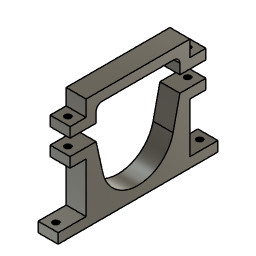
CuadroMediana (Autodesk Fusion 360 design; units mm, degrees)
Autodesk Fusion 360 part; units mm, degrees
sketch "Boceto1" plane through (0, 0, 0) normal (1, 0, 0) x (0, 1, 0)
  line L0 (-17.9997, 45.5) -> (18.0008, 45.5)
  line L1 (21.0003, 42.5) -> (21.0003, 37.5)
  line L2 (21.0003, 37.5) -> (-20.9997, 37.5)
  line L3 (-20.9997, 37.5) -> (-20.9997, 42.5)
  line L4 (-25.9997, 50.5) -> (26.0003, 50.5)
  line L5 (26.0003, 50.5) -> (26.0003, 42.5)
  line L6 (24, 37.5) -> (-27.0128, 37.5)
  line L7 (-25.9997, 42.5) -> (-25.9997, 50.5)
  line L8 (24, 37.5) -> (34.0003, 37.5)
  line L9 (34.0003, 37.5) -> (34.0003, 42.5)
  line L10 (34.0003, 42.5) -> (26.0003, 42.5)
  line L11 (-27.0128, 37.5) -> (-33.9997, 37.5)
  line L12 (-33.9997, 37.5) -> (-33.9997, 42.5)
  line L13 (-33.9997, 42.5) -> (-25.9997, 42.5)
  line L14 (-72.816, 37.5) -> (66.1059, 37.5)
  line L15 (21.0003, 37.5) -> (17.5697, 22.0889)
  line L16 (-20.9997, 37.5) -> (-17.5704, 22.09)
  arc A0 (-17.5704, 22.09) -> (17.5697, 22.0889) centre (-0.0002, 26) ccw
  line L17 (-33.9997, 37.5) -> (-23.996, 37.5)
  line L18 (-25.9997, 32.5) -> (-33.9997, 32.5)
  line L19 (-33.9997, 32.5) -> (-33.9997, 37.5)
  line L20 (24, 37.5) -> (34.0003, 37.5)
  line L21 (34.0003, 37.5) -> (34.0003, 32.5)
  line L22 (34.0003, 32.5) -> (26.0003, 32.5)
  line L23 (-25.9997, 32.5) -> (-25.9997, 7.5)
  line L24 (-25.9997, 7.5) -> (-40, 7.5)
  line L25 (-40, 7.5) -> (-40, 2.5)
  line L26 (-40, 2.5) -> (40.0003, 2.5)
  line L27 (40.0003, 2.5) -> (40.0003, 7.5)
  line L28 (40.0003, 7.5) -> (26.0003, 7.5)
  line L29 (26.0003, 7.5) -> (26.0003, 32.5)
  line L30 (-0.0002, 36.8459) -> (-0.0002, 16.8459)
  arc A1 (-17.9997, 45.5) -> (-20.9997, 42.5) centre (-17.9997, 42.5) ccw
  arc A2 (21.0003, 42.5) -> (17.9998, 45.5) centre (18.0003, 42.5) ccw
  dimension "d3" = 52
  dimension "d6" = 5
  dimension "d8" = 5
  dimension "d13" = 18
  dimension "d16" = 5
  dimension "d18" = 5
  dimension "d19" = 14
  dimension "d20" = 5
  dimension "d23" = 25
  dimension "d25" = 90
  dimension "d26" = 5
  dimension "d27" = 11.5
  dimension "d31" = 3
  dimension "d32" = 3
  dimension "d51" = 42
  dimension "d52" = 5
  dimension "d53" = 8
  dimension "d54" = 8
  dimension "d55" = 52
  dimension "d56" = 8
  dimension "d57" = 13
  dimension "d58" = 8
  dimension "d59" = 14.0003
  dimension "d60" = 8
  constraint horizontal L0
  constraint vertical L1
  constraint horizontal L2
  constraint vertical L3
  constraint horizontal L4
  constraint vertical L5
  constraint horizontal L6
  constraint vertical L7
  constraint horizontal L8
  constraint vertical L9
  constraint horizontal L10
  constraint horizontal L11
  constraint vertical L12
  constraint horizontal L13
  constraint perpendicular L12 L14
  constraint tangent L15 A0
  constraint tangent L16 A0
  constraint horizontal L17
  constraint horizontal L18
  constraint vertical L19
  constraint horizontal L20
  constraint vertical L21
  constraint horizontal L22
  constraint perpendicular L18 L23
  constraint perpendicular L23 L24
  constraint perpendicular L18 L25
  constraint perpendicular L25 L26
  constraint perpendicular L26 L27
  constraint perpendicular L22 L29
  constraint perpendicular L14 L30
  constraint coincident A0.centre L30
  constraint coincident L2.end L14
  constraint coincident L14 L17.end
  constraint tangent L3 A1
  constraint tangent L0 A1
  constraint coincident L0.start A1
  constraint coincident L0 A1.start
  constraint coincident L0.end A2
  constraint tangent L1 A2
  constraint coincident L0 A2.end
  measures "d3" distance of L4.start L4.end
  measures "d6" distance of L8.end L9.end
  measures "d8" distance of L11.end L12.end
  measures "d13" radius of A0
  measures "d16" distance of L11.end L18.end
  measures "d18" distance of L8.end L21.end
  measures "d19" distance of L27.end L28.end
  measures "d20" distance of L26.end L27.end
  measures "d23" distance of L22.end L28.end
  measures "d25" angle of L28 L29
  measures "d26" distance of L24.end L25.end
  measures "d27" distance of L14 A0.centre
  measures "d31" radius of A1
  measures "d32" radius of A2
  measures "d51" distance of L1 L3
  measures "d52" distance of L1 L5
  measures "d53" distance of L9.end L5.end
  measures "d54" distance of L12.end L7.start
  measures "d55" distance of L23 L29
  measures "d56" distance of L18.start L18.end
  measures "d57" distance of L4 L11.end
  measures "d58" distance of L0 L2
  measures "d59" distance of L23.end L24.end
  measures "d60" distance of L21.end L22.end
extrude "Extruir1" add sketch "Boceto1" along normal blind 10 contours L6 L8 L11 L14 L15 L16 A0 L17 L18 L19 L20 L21 L22 L23 L24 L25 L26 L27 L28 L29 makes body 1
move_body "Desplazar1" bodies 1 to x (1, 0, 0) y (0, 1, 0) z (0, 0, 1) at (0, 0, -8)
extrude "Extruir2" add sketch "Boceto1" along normal blind 10 separate body contours L0 L1 L3 L4 L5 L6 L7 L8 L9 L10 L11 L12 L13 L14 L17 L20 A1 A2 makes body 2
sketch "Boceto3" plane through (0, 0, 50.5) normal (0, 0, 1) x (-1, 0, 0)
  line L0 (0, -26.0003) -> (0, 25.9997)
  line L1 (0, 25.9997) -> (-10, 25.9997)
  line L2 (-10, 25.9997) -> (-10, -26.0003)
  line L3 (-10, -26.0003) -> (0, -26.0003)
  line L4 (-10, -40.0003) -> (-10, -26.0003)
  line L5 (0, -34.0003) -> (-10, -34.0003)
  line L6 (0, 33.9997) -> (-10, 33.9997)
  line L7 (0, 40) -> (-10, 40)
  line L8 (0, -40.0003) -> (-10, -40.0003)
  point P0 (-5, 29.9997)
  point P1 (-5, 36)
  point P2 (-5, -30.0003)
  point P3 (-5, -36.0003)
  dimension "d37" = 5
  dimension "d39" = 4
  dimension "d40" = 4
  dimension "d41" = 4
  dimension "d61" = 4
  constraint vertical P0 P1
  constraint vertical P1 P2
  constraint vertical P2 P3
  measures "d37" distance of P3 L4
  measures "d39" distance of L3 P2
  measures "d40" distance of P0 L6
  measures "d41" distance of P1 L7
  measures "d61" distance of P3 L8
hole "Agujero1" at (5, 30.0003, 50.5) at (5, -29.9997, 50.5) direction (0, 0, -1) diameter 2.529 depth 25 tip angle 118 bodies 1 2
thread "Rosca1" "ISO Metric profile 3.0 M3x0.5 6H" major diameter 3.086 minor diameter 2.529 pitch 0.5 angle 60 modelled right hand crest width 0.1368 on face at (3.9733, 29.2621, 28.1667) crest through (6.2645, 30.0003, 29.375) on face at (5.1259, -31.258, 28.1667) crest through (6.2645, -29.9997, 29.375) on face at (5.063, -31.2627, 40.8333) crest through (6.2645, -29.9997, 42.375) on face at (3.9733, 29.2621, 40.8333) crest through (6.2645, 30.0003, 42.375) on bodies 1 2
hole "Agujero2" at (5, 36.0003, 50.5) at (5, -36, 50.5) direction (0, 0, -1) diameter 2.529 end through all bodies 1
thread "Rosca2" "ISO Metric profile 3.0 M3x0.5 6H" major diameter 3.086 minor diameter 2.529 pitch 0.5 angle 60 modelled right hand crest width 0.1368 on face at (3.7359, -36.0315, -2.1667) crest through (6.2645, -36, -0.625) on face at (5.063, 34.7373, -2.1667) crest through (6.2645, 36.0003, -0.625) on bodies 1
